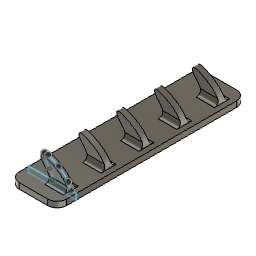
kitchen_hooks (Autodesk Fusion 360 design; units mm, degrees)
Autodesk Fusion 360 part; units mm, degrees
sketch "Sketch1" plane through (0, 0, 0) normal (0, 1, 0) x (1, 0, 0)
  line L0 (-41.0899, -6.2054) -> (8.9101, -6.2054)
  line L1 (8.9101, -6.2054) -> (8.9101, -0.2054)
  line L2 (8.9101, -0.2054) -> (-41.0899, -0.2054)
  line L3 (-41.0899, -0.2054) -> (-41.0899, -6.2054)
  spline S0 degree 5 poles (-16.0899, -6.2054) (-16.0341, -6.5905) (-15.952, -7.352) (-15.9176, -8.4679) (-16.0494, -9.903) (-16.5063, -11.6102) (-17.2409, -13.2342) (-18.2222, -14.783) (-19.3975, -16.2702) (-20.6838, -17.7175) (-21.9745, -19.1499) (-23.1556, -20.5852) (-24.1191, -22.0249) (-24.7769, -23.4448) (-25.0765, -24.785) (-25.0122, -25.9435) (-24.6069, -26.8155) (-23.8987, -27.3238) (-22.9225, -27.4627) (-21.7082, -27.2854) (-20.2846, -26.8691) (-18.6821, -26.2855) (-16.9351, -25.5758) (-15.0807, -24.7609) (-13.1573, -23.8468) (-11.2038, -22.8313) (-9.2586, -21.7102) (-7.3583, -20.4838) (-5.537, -19.1627) (-3.8255, -17.7643) (-2.2516, -16.3101) (-0.8389, -14.8239) (0.3932, -13.3282) (1.4298, -11.8428) (2.2619, -10.381) (2.8846, -8.9506) (3.2138, -7.8344) (3.3657, -7.0136) (3.4248, -6.4736) (3.4439, -6.2054) knots 0 0 0 0 0 0 0.028571 0.057143 0.085714 0.114286 0.142857 0.171429 0.2 0.228571 0.257143 0.285714 0.314286 0.342857 0.371429 0.4 0.428571 0.457143 0.485714 0.514286 0.542857 0.571429 0.6 0.628571 0.657143 0.685714 0.714286 0.742857 0.771429 0.8 0.828571 0.857143 0.885714 0.914286 0.942857 0.971429 1 1 1 1 1 1
  point P0 (-18.7019, -15.3552)
  point P1 (-24.6263, -23.2543)
  point P2 (-24.3442, -26.9217)
  point P3 (-20.5356, -26.9217)
  point P4 (-9.5333, -21.8437)
  point P5 (0.6227, -12.9572)
  dimension "d1" = 50
  dimension "d2" = 6
  constraint horizontal L0
  constraint vertical L1
  constraint horizontal L2
  constraint vertical L3
  constraint midpoint L0 S0.start
  constraint coincident L0 S0.end
  measures "d1" distance of L0.start L0.end
  measures "d2" distance of L0.start L2.end
extrude "Extrude1" add sketch "Sketch1" along normal mid plane 6 contours L0 S0 makes body 1
extrude "Extrude2" add sketch "Sketch1" along normal mid plane 40 contours L0 L1 L2 L3 bodies 1
fillet "Fillet1" radius 5 2 edges at (-6.323, -3, 6.2054) (-6.323, 3, 6.2054) on bodies 1
pattern_linear "R-Pattern1" count 5 spacing 40 along (0, 1, 0) of bodies 1 makes body 2 at (-7.7566, 33.3333, 0.2054) makes body 3 at (-7.7566, 73.3333, 0.2054) makes body 4 at (-7.7566, 113.3333, 0.2054) makes body 5 at (-7.7566, 153.3333, 0.2054)
combine "Combine1" operation add target body 5 tool bodies 4 3 2 1
fillet "Fillet2" radius 10 4 edges at (8.9101, 180, 3.2054) (8.9101, -20, 3.2054) (-41.0899, -20, 3.2054) (-41.0899, 180, 3.2054) on bodies 5
